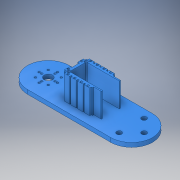
# Autodesk Inventor part: 000.401 - Опорная платформа
Saved by Autodesk Inventor 2019 (Build 230136000, 136)
## iProperties
Created: 2020-03-18
Part Number: 000.401 - Опорная платформа
Material: Пластик АБС
Document SubType Name: Modeling
Designer: Петров Иван
Density: 1.06 g/cm^3
Appearance: Голубой
Author: Петров Иван
Autodesk Inventor part; units mm, degrees
ref_plane "YZ Plane" through (0, 0, 0) normal (1, 0, 0) x (0, 1, 0)
ref_plane "XZ Plane" through (0, 0, 0) normal (0, 1, 0) x (-1, 0, 0)
ref_plane "XY Plane" through (0, 0, 0) normal (0, 0, 1) x (1, 0, 0)
sketch "Эскиз1" plane through (0, 0, 0) normal (0, 1, 0) x (-1, 0, 0)
  circle A0 centre (0, 0) radius 13.8
  circle A1 centre (-8, 0) radius 1.2
  circle A2 centre (0, -8) radius 1.2
  circle A3 centre (8, 0) radius 1.2
  circle A4 centre (0, 8) radius 1.2
  circle A5 centre (-7.7782, 7.7782) radius 1.2813
  circle A6 centre (-11, 0) radius 1.2813
  circle A7 centre (-7.7782, -7.7782) radius 1.2813
  circle A8 centre (0, -11) radius 1.2812
  circle A9 centre (7.7782, -7.7782) radius 1.2812
  circle A10 centre (11, 0) radius 1.2813
  circle A11 centre (7.7782, 7.7782) radius 1.2812
  circle A12 centre (0, 11) radius 1.2812
  circle A13 centre (0, 0) radius 5
  circle A14 centre (0, 0) radius 14
  circle A15 centre (0, 0) radius 1.55
  circle A16 centre (0, 0) radius 1.75
  circle A17 centre (0, 0) radius 25
  dimension "d0" = 50
  constraints: 18 centre point, 1 coincident
  measures "d0" diameter of A17
extrude "Выдавливание1" add sketch "Эскиз1" along normal blind 5 contours A0 | A14 | A17
sketch "Эскиз2" plane through (0, 5, 0) normal (0, 1, 0) x (1, 0, 0)
  line L0 (25, 0) -> (100, 0)
  circle A0 centre (100, 0) radius 25
  line L1 (50, 0) -> (50, -20)
  line L2 (50, 0) -> (50, 20)
  circle A1 centre (0, 0) radius 25 projected
  arc A2 (4.9455, 24.506) -> (95.0545, 24.506) centre (50, 247.5) ccw
  arc A3 (95.0545, -24.506) -> (4.9455, -24.506) centre (50, -247.5) ccw
  line L3 (100, 25) -> (0, 25)
  line L4 (0, -25) -> (100, -25)
  dimension "d3" = 100
  dimension "d4" = 50
  dimension "d5" = 20
  dimension "d6" = 20
  constraints: 15 point on circle, 10 end point, 3 centre point, 3 tangent, 2 vertical, 1 coincident, 1 horizontal, 1 point on line
  measures "d3" distance of point (0, 0) L0.end
  measures "d4" diameter of A0
  measures "d5" distance of L1.start L1.end
  measures "d6" distance of L1.start L2.end
extrude "Выдавливание2" add sketch "Эскиз2" against normal blind 5 contours A1 A2 L2 L0 | L0 L1 A3 A1 | L2 A2 A0 L0 | L0 A0 A3 L1 | A1 L3 A0 A2 | A3 A0 L4 A1 | A0
sketch "Эскиз7" plane through (0, 5, 0) normal (0, 1, 0) x (1, 0, 0)
  line L0 (100, 0) -> (100, 15)
  line L1 (100, 0) -> (100, -15)
  circle A0 centre (100, 15) radius 3
  circle A1 centre (100, -15) radius 3
  line L2 (100, 0) -> (115, 0)
  circle A2 centre (115, 0) radius 3
  point P0 (0, 0)
  dimension "d23" = 15
  dimension "d24" = 15
  dimension "d25" = 6
  dimension "d26" = 6
  dimension "d27" = 15
  dimension "d28" = 6
  constraints: 6 end point, 3 centre point, 3 coincident, 2 vertical, 1 horizontal, 1 other
  measures "d23" distance of L0.start L0.end
  measures "d24" distance of L0.start L1.end
  measures "d25" diameter of A0
  measures "d26" diameter of A1
  measures "d27" distance of L0.start L2.end
  measures "d28" diameter of A2
extrude "Выдавливание7" cut sketch "Эскиз7" against normal blind 10
sketch "Эскиз9" plane through (0, 5, 0) normal (0, 1, 0) x (1, 0, 0)
  line L0 (75.1546, 10) -> (37.0131, 10)
  line L1 (75.1546, 10) -> (75.1546, 11.4565)
  arc A0 (75.1546, 11.4565) -> (74.6046, 11.5) centre (74.6046, 8) ccw
  line L2 (74.6046, 11.5) -> (66.1046, 11.5)
  line L3 (66.1046, 11.5) -> (66.1046, 13)
  line L4 (66.1046, 13) -> (64.6046, 13)
  line L5 (64.6046, 13) -> (64.6046, 15)
  line L6 (64.6046, 15) -> (58.1046, 15)
  line L7 (58.1046, 15) -> (58.1046, 13)
  line L8 (58.1046, 13) -> (56.6046, 13)
  line L9 (56.6046, 13) -> (56.6046, 15)
  line L10 (56.6046, 15) -> (50.1046, 15)
  line L11 (50.1046, 15) -> (50.1046, 13)
  line L12 (50.1046, 13) -> (48.6046, 13)
  line L13 (48.6046, 13) -> (48.6046, 15)
  line L14 (48.6046, 15) -> (42.1046, 15)
  line L15 (42.1046, 15) -> (42.1046, 13)
  line L16 (42.1046, 13) -> (40.6046, 13)
  line L17 (40.6046, 13) -> (40.6046, 15)
  line L18 (40.6046, 15) -> (34.1046, 15)
  line L19 (34.1046, 15) -> (34.1046, 13)
  line L20 (34.1046, 13) -> (32.6046, 13)
  line L21 (32.6046, 13) -> (32.6046, 11.25)
  line L22 (32.6046, 11.25) -> (30.6046, 11.25)
  line L23 (30.6046, 11.25) -> (30.6046, 4.75)
  line L24 (30.6046, 4.75) -> (32.6046, 4.75)
  line L25 (32.6046, 4.75) -> (32.6046, -4.75)
  line L26 (32.6046, -4.75) -> (30.6046, -4.75)
  line L27 (30.6046, -4.75) -> (30.6046, -11.25)
  line L28 (30.6046, -11.25) -> (32.6046, -11.25)
  line L29 (32.6046, -11.25) -> (32.6046, -13)
  line L30 (32.6046, -13) -> (34.1046, -13)
  line L31 (34.1046, -13) -> (34.1046, -15)
  line L32 (34.1046, -15) -> (40.6046, -15)
  line L33 (40.6046, -15) -> (40.6046, -13)
  line L34 (40.6046, -13) -> (42.1046, -13)
  line L35 (42.1046, -13) -> (42.1046, -15)
  line L36 (42.1046, -15) -> (48.6046, -15)
  line L37 (48.6046, -15) -> (48.6046, -13)
  line L38 (48.6046, -13) -> (50.1046, -13)
  line L39 (50.1046, -13) -> (50.1046, -15)
  line L40 (50.1046, -15) -> (56.6046, -15)
  line L41 (56.6046, -15) -> (56.6046, -13)
  line L42 (56.6046, -13) -> (58.1046, -13)
  line L43 (58.1046, -13) -> (58.1046, -15)
  line L44 (58.1046, -15) -> (64.6046, -15)
  line L45 (64.6046, -15) -> (64.6046, -13)
  line L46 (64.6046, -13) -> (66.1046, -13)
  line L47 (66.1046, -13) -> (66.1046, -11.5)
  line L48 (66.1046, -11.5) -> (74.6046, -11.5)
  arc A1 (74.6046, -11.5) -> (75.1267, -11.4608) centre (74.6046, -8) ccw
  line L49 (75.1267, -11.4608) -> (75.1267, -10)
  line L50 (37.0768, -10) -> (75.1267, -10)
  line L51 (37.0768, -10) -> (37.003, -9.9543)
  arc A2 (35.6618, -8.5313) -> (37.003, -9.9543) centre (35.1046, -10.4) ccw
  line L52 (35.6618, -8.5313) -> (35.6046, -8.4256)
  line L53 (35.6046, 8.5152) -> (35.6046, -8.4256)
  arc A3 (37.0131, 10) -> (35.6046, 8.5152) centre (35.1046, 10.4) ccw
  circle A4 centre (53.3546, 13.5) radius 1.25
  circle A5 centre (37.3546, 13.5) radius 1.25
  circle A6 centre (32.1046, -8) radius 1.25
  circle A7 centre (37.3546, -13.5) radius 1.25
  circle A8 centre (45.3546, -13.5) radius 1.25
  circle A9 centre (53.3546, -13.5) radius 1.25
  circle A10 centre (61.3546, -13.5) radius 1.25
  circle A11 centre (32.1046, 8) radius 1.25
  circle A12 centre (45.3546, 13.5) radius 1.25
  circle A13 centre (61.3546, 13.5) radius 1.25
  arc A14 (75.1546, 9.25) -> (77.1046, 7.3) centre (77.1046, 9.25) ccw
  line L54 (75.1546, 9.25) -> (75.1546, 10)
  line L55 (75.1546, 10) -> (59.1546, 10)
  line L56 (59.1546, 10) -> (59.3546, 9.8)
  line L57 (59.3546, 7.0711) -> (59.3546, 9.8)
  arc A15 (59.3546, 7.0711) -> (59.3546, -7.0711) centre (68.1046, 0) ccw
  line L58 (59.3546, -9.8) -> (59.3546, -7.0711)
  line L59 (59.3546, -9.8) -> (59.1546, -10)
  line L60 (59.1546, -10) -> (75.1546, -10)
  line L61 (75.1546, -10) -> (75.1546, -9.25)
  arc A16 (77.1046, -7.3) -> (75.1546, -9.25) centre (77.1046, -9.25) ccw
  line L62 (77.1046, -7.3) -> (78.1046, -7.3)
  line L63 (78.1046, -7.3) -> (78.1046, 7.3)
  line L64 (78.1046, 7.3) -> (77.1046, 7.3)
  circle A17 centre (68.1046, 0) radius 9.1
  line L65 (59.1546, -10) -> (75.1546, -10)
  arc A18 (36.7469, -9.7956) -> (35.805, -8.7963) centre (35.1046, -10.4) ccw
  point P0 (0, 0)
  constraints: 132 end point, 19 centre point, 16 point on circle
extrude "Выдавливание9" add sketch "Эскиз9" along normal blind 28.95 contours L0 A3 L53 L52 A2 L51 L50 L49 A1 L48 L47 L46 L45 L44 L43 L42 L41 L40 L39 L38 L37 L36 L35 L34 L33 L32 L31 L30 L29 L28 L27 L26 L25 L24 L23 L22 L21 L20 L19 L18 L17 L16 L15 L14 L13 L12 L11 L10 L9 L8 L7 L6 L5 L4 L3 L2 A0 L1
equation "\"d6\" = d5"
equation "\"d24\" = d23"
equation "\"d26\" = d25"
equation "\"d27\" = d23"
equation "\"d28\" = d25"
